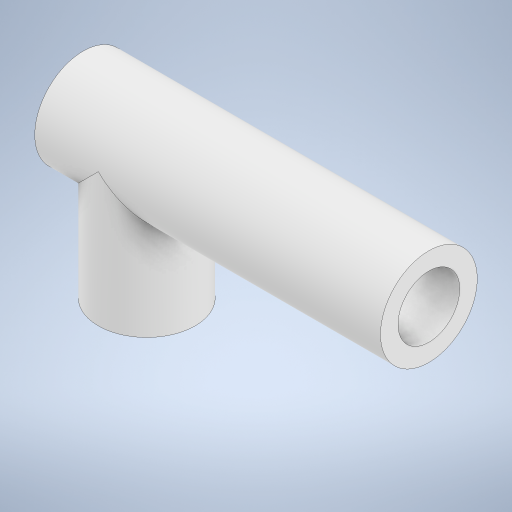
# Autodesk Inventor part: T
Saved by Autodesk Inventor 2024 (Build 280153000, 153)
## iProperties
Created: 2023-02-27
Part Number: T
Material: PVC, no plastificado
Document SubType Name: Modeling
Designer: Braya
Density: 1.29 g/cm^3
Appearance: Suave - Blanco
Mass: 34.8769 g
Surface Area: 178.963 cm^2
Volume: 27.0363 cm^3
Author: Braya
Autodesk Inventor part; units mm, degrees
ref_plane "YZ Plane" through (0, 0, 0) normal (1, 0, 0) x (0, 1, 0)
ref_plane "XZ Plane" through (0, 0, 0) normal (0, 1, 0) x (-1, 0, 0)
sketch "Boceto2" plane through (0, 0, 0) normal (0, 1, 0) x (-1, 0, 0)
  circle A0 centre (0, 0) radius 13.325
  dimension "d0" = 26.65
  constraints: 1 centre point, 1 coincident
  measures "d0" diameter of A0
extrude "Extrusión1" add sketch "Boceto2" along normal blind 36.8
sketch "Boceto3" plane through (0, 0, 0) normal (1, 0, 0) x (0, 1, 0)
  line L0 (0, 0) -> (36.8, 0)
  line L1 (36.8, -13.325) -> (36.8, 13.325) projected
  circle A0 centre (36.8, 0) radius 13.325
  dimension "d11" = 26.65
  constraints: 2 end point, 1 coincident, 1 midpoint, 1 vertical alignment, 2 other
extrude "Extrusión2" add sketch "Boceto3" along normal mid plane 73.14
sketch "Boceto4" plane through (36.57, 36.8, 0) normal (1, 0, 0) x (0, 0, -1)
  circle A0 centre (0, 0) radius 13.325
  point P0 (0, -36.8)
  dimension "d5" = 26.65
  constraints: 1 centre point
  measures "d5" diameter of A0
extrude "Extrusión3" add sketch "Boceto4" along normal blind 41.16
sketch "Boceto5" plane through (0, 0, 0) normal (0, -1, 0) x (1, 0, 0)
  circle A0 centre (0, 0) radius 13.325
  dimension "d8" = 26.65
  constraints: 1 centre point, 1 coincident
  measures "d8" diameter of A0
extrude "Extrusión4" cut sketch "Boceto5" against normal up to surface round surface about axis through (0, 36.8, 0) along (1, 0, 0) radius 13.325 far side no
ref_plane "Plano de trabajo1" through (-17.52, 36.8, 0) normal (-1, 0, 0) x (0, 0, 1)
sketch "Boceto6" plane through (-17.52, 36.8, 0) normal (-1, 0, 0) x (0, 0, 1)
  circle A0 centre (0, 0) radius 13.325 projected
  point P0 (0, -36.8)
extrude "Extrusión5" cut sketch "Boceto6" along normal blind 35.4
sketch "Boceto8" plane through (0, 0, 0) normal (0, -1, 0) x (1, 0, 0)
  circle A0 centre (0, 0) radius 13.325 projected
  circle A1 centre (0, 0) radius 13.325
  constraints: 1 centre point, 1 coincident, 1 concentric
extrude "Extrusión7" add sketch "Boceto8" against normal up to surface round surface about axis through (0, 36.8, 0) along (1, 0, 0) radius 13.325 far side no
sketch "Boceto9" plane through (77.73, 36.8, 0) normal (1, 0, 0) x (0, 0, -1)
  circle A0 centre (0, 0) radius 13.325 projected
  circle A1 centre (0, 0) radius 8.5
  circle A2 centre (0, 0) radius 13.325
  point P0 (0, -36.8)
  dimension "d19" = 17
  dimension "d22" = 26.65
  constraints: 2 centre point, 2 coincident, 1 concentric
  measures "d19" diameter of A1
  measures "d22" diameter of A0
extrude "Extrusión8" cut sketch "Boceto9" against normal blind 109.4225 contours A1
